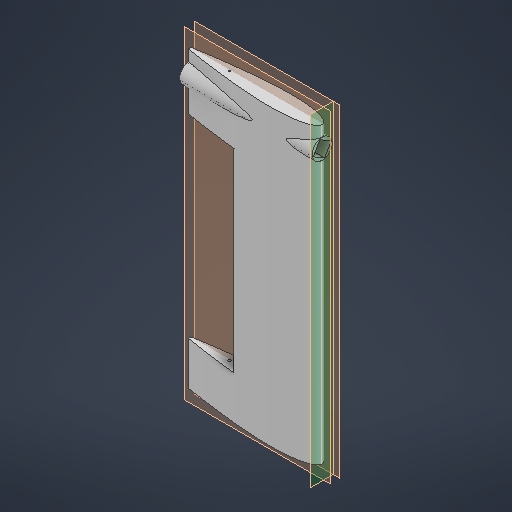
# Autodesk Inventor part: Delb_Tail_v1
Saved by Autodesk Inventor 2026 (Build 300175050, 175E)
## iProperties
Created: 2026-06-09
Part Number: Delb_Tail_v1
Material: Generic
Document SubType Name: Modeling
Designer: Delbe
Density: 1 g/cm^3
Appearance: Default
Author: Delbe
Autodesk Inventor part; units mm, degrees
ref_plane "YZ Plane" through (0, 0, 0) normal (1, 0, 0) x (0, 1, 0)
ref_plane "XZ Plane" through (0, 0, 0) normal (0, 1, 0) x (-1, 0, 0)
ref_plane "XY Plane" through (0, 0, 0) normal (0, 0, 1) x (1, 0, 0)
sketch "Sketch5" plane through (0, 0, 0) normal (0, 1, 0) x (-1, 0, 0)
  spline S0 degree 4 poles (214, 0.3449) (213.9235, 0.3586) (213.5504, 0.4255) (212.9247, 0.5375) (211.8694, 0.7251) (210.7617, 0.9209) (209.4043, 1.1592) (207.8102, 1.4368) (205.9789, 1.7525) (203.9169, 2.1042) (201.6282, 2.4897) (199.1185, 2.907) (196.3936, 3.3535) (193.4599, 3.8269) (190.3242, 4.3245) (186.9939, 4.8439) (183.4768, 5.3823) (179.781, 5.937) (175.9152, 6.5054) (171.8885, 7.0847) (167.7102, 7.6721) (163.3902, 8.265) (158.9384, 8.8603) (154.3653, 9.4553) (149.6816, 10.047) (144.8982, 10.6323) (140.0263, 11.2083) (135.0773, 11.7717) (130.0627, 12.3193) (124.9942, 12.8478) (119.8837, 13.3538) (114.7431, 13.8337) (109.5844, 14.2841) (104.4196, 14.7015) (99.2609, 15.0822) (94.1202, 15.4227) (89.0095, 15.7197) (83.9407, 15.9697) (78.9258, 16.1695) (73.9764, 16.3162) (69.104, 16.4071) (64.32, 16.4396) (59.6357, 16.4118) (55.0618, 16.3218) (50.6091, 16.1683) (46.288, 15.9504) (42.1085, 15.6678) (38.0804, 15.3204) (34.213, 14.9088) (30.5154, 14.4338) (26.9962, 13.8969) (23.6634, 13.3) (20.5248, 12.6451) (17.5876, 11.9348) (14.8584, 11.1717) (12.3433, 10.3589) (10.0479, 9.4991) (7.977, 8.5956) (6.1348, 7.651) (4.5247, 6.6676) (3.1496, 5.6471) (2.0123, 4.5896) (1.1163, 3.495) (0.468, 2.3618) (0.0758, 1.1958) (-0.0534, 0) (0.0758, -1.1958) (0.468, -2.3618) (1.1163, -3.495) (2.0123, -4.5896) (3.1496, -5.6471) (4.5247, -6.6676) (6.1348, -7.651) (7.977, -8.5956) (10.0479, -9.4991) (12.3433, -10.3589) (14.8584, -11.1717) (17.5876, -11.9348) (20.5248, -12.6451) (23.6634, -13.3) (26.9962, -13.8969) (30.5154, -14.4338) (34.213, -14.9088) (38.0804, -15.3204) (42.1085, -15.6678) (46.288, -15.9504) (50.6091, -16.1683) (55.0618, -16.3218) (59.6357, -16.4118) (64.32, -16.4396) (69.104, -16.4071) (73.9764, -16.3162) (78.9258, -16.1695) (83.9407, -15.9697) (89.0095, -15.7197) (94.1202, -15.4227) (99.2609, -15.0822) (104.4196, -14.7015) (109.5844, -14.2841) (114.7431, -13.8337) (119.8837, -13.3538) (124.9942, -12.8478) (130.0627, -12.3193) (135.0773, -11.7717) (140.0263, -11.2083) (144.8982, -10.6323) (149.6816, -10.047) (154.3653, -9.4553) (158.9384, -8.8603) (163.3902, -8.265) (167.7102, -7.6721) (171.8885, -7.0847) (175.9152, -6.5054) (179.781, -5.937) (183.4768, -5.3823) (186.9939, -4.8439) (190.3242, -4.3245) (193.4599, -3.8269) (196.3936, -3.3535) (199.1185, -2.907) (201.6282, -2.4897) (203.9169, -2.1042) (205.9789, -1.7525) (207.8102, -1.4368) (209.4043, -1.1592) (210.7617, -0.9209) (211.8694, -0.7251) (212.9247, -0.5375) (213.5504, -0.4255) (213.9235, -0.3586) (214, -0.3449) knots 0 0 0 0 0 0.006275 0.009968 0.014263 0.019074 0.024344 0.030027 0.036088 0.042498 0.04923 0.056263 0.063574 0.071147 0.078961 0.087003 0.095255 0.103702 0.112331 0.121128 0.130079 0.13917 0.148391 0.157726 0.167166 0.176696 0.186306 0.195983 0.205715 0.215491 0.225299 0.235127 0.244964 0.254798 0.264619 0.274414 0.284172 0.293881 0.303532 0.313111 0.322608 0.332012 0.34131 0.350493 0.359549 0.368466 0.377233 0.385838 0.39427 0.402518 0.410569 0.418411 0.426034 0.433424 0.440569 0.447459 0.454083 0.460432 0.466498 0.472281 0.477786 0.483031 0.48805 0.4929 0.497646 0.502354 0.5071 0.51195 0.516969 0.522214 0.527719 0.533502 0.539568 0.545917 0.552541 0.559431 0.566576 0.573966 0.581589 0.589431 0.597482 0.60573 0.614162 0.622767 0.631534 0.640451 0.649507 0.65869 0.667988 0.677392 0.686889 0.696468 0.706119 0.715828 0.725586 0.735381 0.745202 0.755036 0.764873 0.774701 0.784509 0.794285 0.804017 0.813694 0.823304 0.832834 0.842274 0.851609 0.86083 0.869921 0.878872 0.887669 0.896298 0.904745 0.912997 0.921039 0.928853 0.936426 0.943737 0.95077 0.957502 0.963912 0.969973 0.975656 0.980926 0.985737 0.990032 0.993725 1 1 1 1 1
  line L0 (204.525, -2) -> (204.525, 2)
  line L1 (204.525, 0) -> (0, 0)
  line L2 (0, 0) -> (61.2, 0)
  line L3 (61.2, 0) -> (61.2, -16.415)
  line L4 (61.2, -16.415) -> (61.2, 16.415)
  point P0 (0, 0)
  point P1 (213.875, 0.3673)
  point P2 (213.5005, 0.4344)
  point P3 (212.8772, 0.5457)
  point P4 (212.0066, 0.7006)
  point P5 (210.8908, 0.8979)
  point P6 (209.5323, 1.1364)
  point P7 (207.9344, 1.4146)
  point P8 (206.1007, 1.7309)
  point P9 (204.0356, 2.0831)
  point P10 (201.7438, 2.4693)
  point P11 (199.2308, 2.8872)
  point P12 (196.5023, 3.3344)
  point P13 (193.5648, 3.8084)
  point P14 (190.4252, 4.3068)
  point P15 (187.0907, 4.8269)
  point P16 (183.5691, 5.366)
  point P17 (179.8687, 5.9215)
  point P18 (175.9981, 6.4907)
  point P19 (171.9664, 7.0708)
  point P20 (167.7829, 7.6591)
  point P21 (163.4575, 8.2526)
  point P22 (159.0002, 8.8488)
  point P23 (154.4215, 9.4444)
  point P24 (149.732, 10.0368)
  point P25 (144.9427, 10.6228)
  point P26 (140.0648, 11.1993)
  point P27 (135.1097, 11.7633)
  point P28 (130.0889, 12.3114)
  point P29 (125.0142, 12.8402)
  point P30 (119.8974, 13.3464)
  point P31 (114.7505, 13.8266)
  point P32 (109.5855, 14.2771)
  point P33 (104.4145, 14.6943)
  point P34 (99.2495, 15.0749)
  point P35 (94.1026, 15.4151)
  point P36 (88.9858, 15.7116)
  point P37 (83.9111, 15.961)
  point P38 (78.8903, 16.1601)
  point P39 (73.9352, 16.306)
  point P40 (69.0573, 16.3958)
  point P41 (64.268, 16.4271)
  point P42 (59.5785, 16.3978)
  point P43 (54.9998, 16.3062)
  point P44 (50.5425, 16.1509)
  point P45 (46.2171, 15.931)
  point P46 (42.0336, 15.6461)
  point P47 (38.0019, 15.2962)
  point P48 (34.1313, 14.8818)
  point P49 (30.4309, 14.4038)
  point P50 (26.9093, 13.8636)
  point P51 (23.5748, 13.2629)
  point P52 (20.4352, 12.6039)
  point P53 (17.4977, 11.889)
  point P54 (14.7693, 11.1209)
  point P55 (12.2562, 10.3027)
  point P56 (9.9644, 9.4372)
  point P57 (7.8993, 8.5276)
  point P58 (6.0656, 7.5769)
  point P59 (4.4677, 6.5883)
  point P60 (3.1092, 5.5644)
  point P61 (1.9934, 4.5081)
  point P62 (1.1228, 3.4216)
  point P63 (0.4995, 2.307)
  point P64 (0.125, 1.1661)
  point P65 (0.125, -1.1661)
  point P66 (0.4995, -2.307)
  point P67 (1.1228, -3.4216)
  point P68 (1.9934, -4.5081)
  point P69 (3.1092, -5.5644)
  point P70 (4.4677, -6.5883)
  point P71 (6.0656, -7.5769)
  point P72 (7.8993, -8.5276)
  point P73 (9.9644, -9.4372)
  point P74 (12.2562, -10.3027)
  point P75 (14.7693, -11.1209)
  point P76 (17.4977, -11.889)
  point P77 (20.4352, -12.6039)
  point P78 (23.5748, -13.2629)
  point P79 (26.9093, -13.8636)
  point P80 (30.4309, -14.4038)
  point P81 (34.1313, -14.8818)
  point P82 (38.0019, -15.2962)
  point P83 (42.0336, -15.6461)
  point P84 (46.2171, -15.931)
  point P85 (50.5425, -16.1509)
  point P86 (54.9998, -16.3062)
  point P87 (59.5785, -16.3978)
  point P88 (64.268, -16.4271)
  point P89 (69.0573, -16.3958)
  point P90 (73.9352, -16.306)
  point P91 (78.8903, -16.1601)
  point P92 (83.9111, -15.961)
  point P93 (88.9858, -15.7116)
  point P94 (94.1026, -15.4151)
  point P95 (99.2495, -15.0749)
  point P96 (104.4145, -14.6943)
  point P97 (109.5855, -14.2771)
  point P98 (114.7505, -13.8266)
  point P99 (119.8974, -13.3464)
  point P100 (125.0142, -12.8402)
  point P101 (130.0889, -12.3114)
  point P102 (135.1097, -11.7633)
  point P103 (140.0648, -11.1993)
  point P104 (144.9427, -10.6228)
  point P105 (149.732, -10.0368)
  point P106 (154.4215, -9.4444)
  point P107 (159.0002, -8.8488)
  point P108 (163.4575, -8.2526)
  point P109 (167.7829, -7.6591)
  point P110 (171.9664, -7.0708)
  point P111 (175.9981, -6.4907)
  point P112 (179.8687, -5.9215)
  point P113 (183.5691, -5.366)
  point P114 (187.0907, -4.8269)
  point P115 (190.4252, -4.3068)
  point P116 (193.5648, -3.8084)
  point P117 (196.5023, -3.3344)
  point P118 (199.2308, -2.8872)
  point P119 (201.7438, -2.4693)
  point P120 (204.0356, -2.0831)
  point P121 (206.1007, -1.7309)
  point P122 (207.9344, -1.4146)
  point P123 (209.5323, -1.1364)
  point P124 (210.8908, -0.8979)
  point P125 (212.0066, -0.7006)
  point P126 (212.8772, -0.5457)
  point P127 (213.5005, -0.4344)
  point P128 (213.875, -0.3673)
  dimension "d28" = 204.525
  dimension "d29" = 61.2
  dimension "d30" = 32.8299
  constraints: 10 end point, 2 point on line, 1 horizontal, 1 midpoint, 1 perpendicular, 1 vertical, 135 other
  measures "d28" distance of L1.start L1.end
  measures "d29" distance of L1.end L2.end
  measures "d30" distance of L3.end L4.end
extrude "Main Wing" add sketch "Sketch5" along normal blind 453.491
sketch "Sketch6" plane through (-204.525, 0, 2) normal (-1, 0, 0) x (0, 0, 1)
  line L0 (0, 0) -> (0, 66.548)
  line L1 (0, 453.4889) -> (0, 366.5701)
  line L2 (20, 366.5701) -> (-20, 366.5701)
  line L3 (-20, 66.548) -> (20, 66.548)
  line L4 (20, 66.548) -> (20, 366.5701)
  line L5 (-20, 366.5701) -> (-20, 66.548)
  point P0 (-2, 0)
  dimension "d31" = 66.548
  dimension "d32" = 86.9188
  dimension "d33" = 40
  dimension "d34" = 40
  dimension "d43" = 300.0221
  constraints: 12 end point, 3 vertical, 2 horizontal, 2 midpoint
  measures "d31" distance of L0.start L0.end
  measures "d32" distance of L1.start L1.end
  measures "d33" distance of L2.start L2.end
  measures "d34" distance of L3.start L3.end
  measures "d43" distance of L3.end L2.start
extrude "Rectangle Elevron Gap" cut sketch "Sketch6" against normal blind 69.6214
sketch "Sketch7" plane through (-204.525, 66.548, 2) normal (0, 1, 0) x (1, 0, 0)
  line L0 (69.6201, 13.7865) -> (69.6201, -9.7851)
  line L1 (69.6201, -9.7851) -> (69.6201, 2.0009)
  circle A0 centre (69.6201, 2.0009) radius 17
  circle A1 centre (69.6201, 2.0009) radius 1.7526
  point P0 (204.525, 2)
  point P1 (69.6201, 3.7535)
  point P2 (69.6201, 0.2483)
  dimension "d37" = 23.5717
  dimension "d38" = 11.786
  dimension "d41" = 34
  dimension "d42" = 3.5052
  constraints: 4 end point, 2 centre point, 1 coincident, 1 point on line, 1 vertical
  measures "d37" distance of L0.start L0.end
  measures "d38" distance of L0.end L1.end
  measures "d41" diameter of A0
  measures "d42" diameter of A1
extrude "Circle Elevron Gap" cut sketch "Sketch7" along normal blind 300.0221 contours A1 L0 | A0 picked at (69.7501, 0.8471)
sketch "Sketch8" plane through (0, 453.491, 0) normal (0, 1, 0) x (1, 0, 0)
  line L0 (-204.5238, 0) -> (-143.0304, 0)
  circle A0 centre (-143.0304, 0) radius 1.7526
  point P0 (0, 0)
  dimension "d46" = 61.4934
  dimension "d47" = 3.5052
  constraints: 2 end point, 1 centre point, 1 coincident, 1 horizontal
  measures "d46" distance of L0.start L0.end
  measures "d47" diameter of A0
extrude "Elevron Screw Hole" cut sketch "Sketch8" against normal blind 454.0221
ref_plane "Leading Edge Plane" through (0, 226.7455, 0) normal (-1, 0, 0) x (0, 0, 1)
sketch "Sketch9" plane through (0, 226.7455, 0) normal (-1, 0, 0) x (0, 0, 1)
  line L0 (0, -226.7455) -> (0, 226.7401)
  line L1 (0, 226.7401) -> (0, 213.1781)
  line L2 (0, 213.1781) -> (0, 194.4281)
  circle A0 centre (0, 194.4281) radius 18.75
  line L3 (-14.0018, 198.1799) -> (3.7518, 208.4299)
  line L4 (3.7518, 208.4299) -> (14.0018, 190.6764)
  line L5 (14.0018, 190.6764) -> (-3.7518, 180.4264)
  line L6 (-3.7518, 180.4264) -> (-14.0018, 198.1799)
  line L7 (-14.0018, 198.1799) -> (14.0018, 190.6764) construction
  line L8 (3.7518, 208.4299) -> (-3.7518, 180.4264) construction
  circle A1 centre (0, 194.4281) radius 15.5
  dimension "d50" = 13.562
  dimension "d51" = 18.75
  dimension "d52" = 37.5
  dimension "d55" = 20.5
  dimension "d56" = 20.5
  dimension "d70" = 31
  constraints: 18 end point, 2 centre point, 2 coincident, 2 midpoint, 2 parallel, 2 point on line, 1 perpendicular, 1 vertical
  measures "d50" distance of L0.end L1.end
  measures "d51" distance of L1.end L2.end
  measures "d52" diameter of A0
  measures "d55" distance of L4.end L5.end
  measures "d56" distance of L3.end L4.end
  measures "d70" diameter of A1
extrude "Circle thingy for boom" add sketch "Sketch9" along normal blind 204.5 contours A1 L0 L3 L6 L5 | L0 L5 L4 L3 A1 | L5 L6 L3 L0 | L0 L3 L4 L5
sketch "Sketch10" plane through (0, 226.7455, 0) normal (1, 0, 0) x (0, 0, -1)
  line L0 (0, 213.1791) -> (0, 194.4291)
  line L1 (14.0018, 198.1809) -> (-3.7518, 208.4309)
  line L2 (-3.7518, 208.4309) -> (-14.0018, 190.6773)
  line L3 (-14.0018, 190.6773) -> (3.7518, 180.4273)
  line L4 (3.7518, 180.4273) -> (14.0018, 198.1809)
  line L5 (14.0018, 198.1809) -> (-14.0018, 190.6773) construction
  line L6 (-3.7518, 208.4309) -> (3.7518, 180.4273) construction
  point P0 (0, -226.7455)
  dimension "d57" = 18.75
  dimension "d58" = 20.5
  dimension "d59" = 20.5
  constraints: 14 end point, 2 parallel, 1 perpendicular, 1 vertical
  measures "d57" distance of L0.start L0.end
  measures "d58" distance of L3.end L2.end
  measures "d59" distance of L2.end L1.end
extrude "20x20 hole for boom" cut sketch "Sketch10" against normal blind 205.5
ref_plane "Plane of Pain" through (-204.525, 0, -17) normal (0, 0, 1) x (0, 1, 0)
ref_plane "Work Plane5" through (-204.525, 0, -2) normal (0, 0, 1) x (0, 1, 0)
sketch "Sketch11" plane through (-204.525, 0, -17) normal (0, 0, 1) x (0, 1, 0)
  line L0 (453.4842, 0.0013) -> (403.4842, 0.0013)
  line L1 (403.4842, 0.0013) -> (404.7122, -149.9936)
  circle A0 centre (404.7122, -149.9936) radius 5.25
  line L2 (404.7122, -149.9936) -> (219.7122, -149.9936)
  circle A1 centre (219.7122, -149.9936) radius 5.25
  point P0 (0, -204.525)
  dimension "d64" = 50
  dimension "d65" = 150
  dimension "d66" = 10.5
  dimension "d67" = 185
  constraints: 6 end point, 2 centre point, 2 coincident, 2 horizontal, 1 equal radius
  measures "d64" distance of L0.start L0.end
  measures "d65" distance of L0.end L1.end
  measures "d66" diameter of A0
  measures "d67" distance of L2.start L2.end
extrude "Some screw holes" cut sketch "Sketch11" along normal blind 5.25
body "Solid3"
